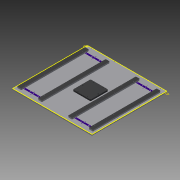
# Autodesk Inventor part: Top_part
Saved by Autodesk Inventor 2015 SP2 (Build 190223200, 223)
## iProperties
Created: 2016-11-11
Part Number: Top_part
Material: Generic
Document SubType Name: Modeling
Designer: Yann Cesbron
Density: 1 g/cm^3
Appearance: Default
Mass: 3815.36 g
Surface Area: 8876.44 cm^2
Volume: 3815.36 cm^3
Material: Perspex Black 9961 -10 mm
Author: Yann Cesbron
Autodesk Inventor part; units mm, degrees
ref_plane "YZ Plane" through (0, 0, 0) normal (1, 0, 0) x (0, 1, 0)
ref_plane "XZ Plane" through (0, 0, 0) normal (0, 1, 0) x (-1, 0, 0)
ref_plane "XY Plane" through (0, 0, 0) normal (0, 0, 1) x (1, 0, 0)
ref_plane "Work Plane2" through (0, 0, 0) normal (0, 0, 1) x (1, 0, 0)
sketch "Sketch2" plane through (0, 0, 0) normal (0, 0, 1) x (1, 0, 0)
  line L0 (-10, 10) -> (575, 10)
  line L1 (575, 10) -> (575, -540)
  line L2 (575, -540) -> (-10, -540)
  line L3 (-10, -540) -> (-10, 10)
  point P0 (0, 0)
  dimension "d0" = 585
  dimension "d1" = 550
  dimension "d3" = 10
  dimension "d10" = 10
  constraints: 8 end point, 2 parallel, 1 horizontal, 1 perpendicular
  measures "d0" distance of L1.end L2.end
  measures "d1" distance of L0.end L1.end
  measures "d3" distance from line of point (0, 0) L0
  measures "d10" distance from line of L3 point (0, 0)
extrude "Extrusion1" add sketch "Sketch2" along normal blind 10
sketch "Cut_out_top" plane through (0, 0, 10) normal (0, 0, 1) x (1, 0, 0)
  line L0 (340, -320) -> (250, -320)
  line L1 (245, -315) -> (245, -225)
  line L2 (250, -220) -> (340, -220)
  line L3 (345, -225) -> (345, -315)
  line L4 (345, -320) -> (245, -220) construction
  line L5 (245, -320) -> (345, -220) construction
  line L6 (575, 10) -> (-10, 10) projected
  line L7 (575, -540) -> (575, 10) projected
  line L8 (548, -510) -> (545, -510)
  line L9 (545, -510) -> (545, -30)
  line L10 (545, -30) -> (548, -30)
  line L11 (548, -30) -> (548, -510)
  line L12 (-10, -540) -> (575, -540) projected
  line L13 (173, -510) -> (170, -510)
  line L14 (170, -510) -> (170, -30)
  line L15 (170, -30) -> (173, -30)
  line L16 (173, -30) -> (173, -510)
  line L17 (17, -30) -> (20, -30)
  line L18 (20, -510) -> (17, -510)
  line L19 (17, -510) -> (17, -30)
  line L20 (20, -30) -> (20, -510)
  line L21 (392, -30) -> (395, -30)
  line L22 (395, -510) -> (392, -510)
  line L23 (392, -510) -> (392, -30)
  line L24 (395, -30) -> (395, -510)
  line L25 (-10, 10) -> (-10, -540) projected
  circle A0 centre (260, -327.5) radius 1.65
  circle A1 centre (330, -327.5) radius 1.65
  circle A2 centre (330, -212.5) radius 1.65
  circle A3 centre (260, -212.5) radius 1.65
  circle A4 centre (352.5, -270) radius 2.5
  circle A5 centre (237.5, -270) radius 2.5
  circle A6 centre (520, -496) radius 2.25
  circle A7 centre (420, -496) radius 2.25
  circle A8 centre (145, -496) radius 2.25
  circle A9 centre (45, -496) radius 2.25
  circle A10 centre (45, -44) radius 2.25
  circle A11 centre (145, -44) radius 2.25
  circle A12 centre (520, -44) radius 2.25
  circle A13 centre (420, -44) radius 2.25
  circle A14 centre (538, -481) radius 1.65
  circle A15 centre (538, -59) radius 1.65
  circle A16 centre (555, -411) radius 1.65
  circle A17 centre (538, -341) radius 1.65
  circle A18 centre (538, -199) radius 1.65
  circle A19 centre (555, -270) radius 1.65
  circle A20 centre (555, -129) radius 1.65
  circle A21 centre (402, -481) radius 1.65
  circle A22 centre (385, -411) radius 1.65
  circle A23 centre (402, -341) radius 1.65
  circle A24 centre (385, -270) radius 1.65
  circle A25 centre (402, -199) radius 1.65
  circle A26 centre (385, -129) radius 1.65
  circle A27 centre (402, -59) radius 1.65
  circle A28 centre (163, -481) radius 1.65
  circle A29 centre (180, -411) radius 1.65
  circle A30 centre (163, -341) radius 1.65
  circle A31 centre (180, -270) radius 1.65
  circle A32 centre (163, -199) radius 1.65
  circle A33 centre (180, -129) radius 1.65
  circle A34 centre (163, -59) radius 1.65
  circle A35 centre (27, -481) radius 1.65
  circle A36 centre (10, -411) radius 1.65
  circle A37 centre (27, -341) radius 1.65
  circle A38 centre (10, -270) radius 1.65
  circle A39 centre (27, -199) radius 1.65
  circle A40 centre (10, -129) radius 1.65
  circle A41 centre (27, -59) radius 1.65
  arc A42 (340, -320) -> (345, -315) centre (340, -315) ccw
  arc A43 (245, -315) -> (250, -320) centre (250, -315) ccw
  arc A44 (250, -220) -> (245, -225) centre (250, -225) ccw
  arc A45 (345, -225) -> (340, -220) centre (340, -225) ccw
  circle A46 centre (535, 5) radius 2.25
  circle A47 centre (370, 5) radius 2.25
  circle A48 centre (195, 5) radius 2.25
  circle A49 centre (30, 5) radius 2.25
  circle A50 centre (-5, -25) radius 2.25
  circle A51 centre (-5, -505) radius 2.25
  circle A52 centre (-5, -185) radius 2.25
  circle A53 centre (-5, -345) radius 2.25
  circle A54 centre (570, -25) radius 2.25
  circle A55 centre (570, -505) radius 2.25
  circle A56 centre (570, -345) radius 2.25
  circle A57 centre (570, -185) radius 2.25
  point P0 (0, 0)
  point P1 (295, -270)
  dimension "d6" = 100
  dimension "d7" = 100
  dimension "d8" = 280
  dimension "d9" = 280
  dimension "d49" = 3
  dimension "d50" = 480
  dimension "d53" = 3
  dimension "d54" = 480
  dimension "d55" = 3
  dimension "d56" = 480
  dimension "d57" = 3
  dimension "d58" = 480
  dimension "d59" = 30
  dimension "d60" = 30
  dimension "d61" = 30
  dimension "d62" = 150
  dimension "d63" = 30
  dimension "d64" = 30
  dimension "d65" = 30
  dimension "d66" = 150
  dimension "d94" = 3.3
  dimension "d95" = 3.3
  dimension "d96" = 3.3
  dimension "d97" = 3.3
  dimension "d98" = 15
  dimension "d99" = 15
  dimension "d100" = 15
  dimension "d101" = 15
  dimension "d102" = 7.5
  dimension "d103" = 7.5
  dimension "d104" = 7.5
  dimension "d105" = 7.5
  dimension "d106" = 245
  dimension "d111" = 5
  dimension "d112" = 5
  dimension "d113" = 7.5
  dimension "d114" = 7.5
  dimension "d115" = 50
  dimension "d116" = 50
  dimension "d132" = 4.5
  dimension "d133" = 4.5
  dimension "d134" = 4.5
  dimension "d135" = 4.5
  dimension "d136" = 4.5
  dimension "d137" = 4.5
  dimension "d138" = 4.5
  dimension "d139" = 4.5
  dimension "d147" = 55
  dimension "d148" = 44
  dimension "d149" = 44
  dimension "d150" = 100
  dimension "d151" = 55
  dimension "d152" = 44
  dimension "d153" = 100
  dimension "d154" = 44
  dimension "d155" = 54
  dimension "d156" = 54
  dimension "d157" = 55
  dimension "d158" = 100
  dimension "d159" = 55
  dimension "d160" = 54
  dimension "d161" = 54
  dimension "d162" = 100
  dimension "d163" = 3.3
  constraints: 58 centre point, 44 end point, 10 parallel, 8 point on circle, 8 point on line, 8 tangent, 5 horizontal, 5 perpendicular, 2 equal radius, 2 midpoint
  measures "d6" distance of L4.end L5.end
  measures "d7" distance of L5.start L4.end
  measures "d8" distance from line of L6 point (295, -270)
  measures "d9" distance from line of L7 point (295, -270)
  measures "d49" distance of L9.end L10.end
  measures "d50" distance of L8.end L9.end
  measures "d53" distance of L15.start L15.end
  measures "d54" distance of L13.end L15.start
  measures "d55" distance of L17.start L17.end
  measures "d56" distance of L19.start L17.start
  measures "d57" distance of L21.start L21.end
  measures "d58" distance of L23.start L21.start
  measures "d59" distance between parallel lines of L7 L9
  measures "d60" distance between parallel lines of L12 L8
  measures "d61" distance between parallel lines of L12 L22
  measures "d62" distance between parallel lines of L24 L9
  measures "d63" distance between parallel lines of L12 L18
  measures "d64" distance between parallel lines of L25 L20
  measures "d65" distance between parallel lines of L12 L13
  measures "d66" distance between parallel lines of L14 L20
  measures "d94" diameter of A0
  measures "d95" diameter of A1
  measures "d96" diameter of A2
  measures "d97" diameter of A3
  measures "d98" distance from line of L1 A0.centre
  measures "d99" distance from line of L3 A1.centre
  measures "d100" distance from line of L1 A3.centre
  measures "d101" distance from line of L3 A2.centre
  measures "d102" distance from line of L0 A1.centre
  measures "d103" distance from line of L0 A0.centre
  measures "d104" distance from line of L2 A3.centre
  measures "d105" distance from line of L2 A2.centre
  measures "d106" distance from line of L7 A1.centre
  measures "d111" diameter of A4
  measures "d112" diameter of A5
  measures "d113" distance from line of L3 A4.centre
  measures "d114" distance from line of L1 A5.centre
  measures "d115" distance from line of L0 A4.centre
  measures "d116" distance from line of L0 A5.centre
  measures "d132" diameter of A6
  measures "d133" diameter of A7
  measures "d134" diameter of A8
  measures "d135" diameter of A9
  measures "d136" diameter of A10
  measures "d137" diameter of A11
  measures "d138" diameter of A12
  measures "d139" diameter of A13
  measures "d147" distance from line of L7 A6.centre
  measures "d148" distance from line of L12 A6.centre
  measures "d149" distance from line of L12 A7.centre
  measures "d150" distance of A6.centre A7.centre
  measures "d151" distance from line of L25 A9.centre
  measures "d152" distance from line of L12 A9.centre
  measures "d153" distance of A8.centre A9.centre
  measures "d154" distance from line of L12 A8.centre
  measures "d155" distance from line of L6 A10.centre
  measures "d156" distance from line of L6 A11.centre
  measures "d157" distance from line of L25 A10.centre
  measures "d158" distance of A11.centre A10.centre
  measures "d159" distance from line of L7 A12.centre
  measures "d160" distance from line of L6 A13.centre
  measures "d161" distance from line of L6 A12.centre
  measures "d162" distance of A13.centre A12.centre
  measures "d163" diameter of A14
sketch "Air_duct_attachment_top" plane through (0, 0, 10) normal (0, 0, 1) x (1, 0, 0)
  line L0 (545, -500) -> (395, -500)
  line L1 (395, -500) -> (395, -492)
  line L2 (395, -492) -> (545, -492)
  line L3 (545, -492) -> (545, -500)
  line L4 (420, -496) -> (520, -496)
  circle A0 centre (520, -496) radius 1.65
  circle A1 centre (420, -496) radius 1.65
  line L5 (575, -540) -> (575, 10) projected
  line L6 (170, -500) -> (20, -500)
  line L7 (20, -500) -> (20, -492)
  line L8 (20, -492) -> (170, -492)
  line L9 (170, -492) -> (170, -500)
  line L10 (45, -496) -> (145, -496)
  circle A2 centre (145, -496) radius 1.65
  circle A3 centre (45, -496) radius 1.65
  line L11 (-10, -540) -> (575, -540) projected
  line L12 (545, -48) -> (395, -48)
  line L13 (395, -48) -> (395, -40)
  line L14 (395, -40) -> (545, -40)
  line L15 (545, -40) -> (545, -48)
  line L16 (420, -44) -> (520, -44)
  circle A4 centre (520, -44) radius 1.65
  circle A5 centre (420, -44) radius 1.65
  line L17 (170, -40) -> (170, -48)
  circle A6 centre (145, -44) radius 1.65
  line L18 (45, -44) -> (145, -44)
  line L19 (170, -48) -> (20, -48)
  line L20 (20, -40) -> (170, -40)
  circle A7 centre (45, -44) radius 1.65
  line L21 (20, -48) -> (20, -40)
  line L22 (-10, -540) -> (-10, 10) projected
  line L23 (575, 10) -> (-10, 10) projected
  point P0 (0, 0)
  point P1 (470, -496)
  point P2 (470, -496)
  point P3 (95, -496)
  point P4 (95, -496)
  point P5 (470, -44)
  point P6 (470, -44)
  point P7 (95, -44)
  point P8 (95, -44)
  dimension "d11" = 150
  dimension "d12" = 8
  dimension "d15" = 100
  dimension "d20" = 3.3
  dimension "d21" = 25
  dimension "d23" = 3.3
  dimension "d24" = 105
  dimension "d25" = 150
  dimension "d26" = 8
  dimension "d27" = 100
  dimension "d28" = 3.3
  dimension "d29" = 25
  dimension "d30" = 3.3
  dimension "d32" = 40
  dimension "d33" = 150
  dimension "d34" = 8
  dimension "d35" = 100
  dimension "d36" = 3.3
  dimension "d37" = 25
  dimension "d38" = 3.3
  dimension "d39" = 150
  dimension "d40" = 8
  dimension "d41" = 100
  dimension "d42" = 3.3
  dimension "d43" = 25
  dimension "d44" = 3.3
  dimension "d45" = 40
  dimension "d46" = 105
  dimension "d47" = 105
  dimension "d48" = 105
  dimension "d68" = 50
  dimension "d69" = 50
  constraints: 40 end point, 12 coincident, 12 parallel, 8 centre point, 4 horizontal, 4 midpoint, 4 perpendicular, 4 other
  measures "d11" distance of L1.end L2.end
  measures "d12" distance of L0.end L1.end
  measures "d15" distance of L4.end L4.start
  measures "d20" diameter of A1
  measures "d21" distance from line of L3 L4.end
  measures "d23" diameter of A0
  measures "d24" distance from line of L5 point (470, -496)
  measures "d25" distance of L7.end L8.end
  measures "d26" distance of L6.end L7.end
  measures "d27" distance of L10.end L10.start
  measures "d28" diameter of A3
  measures "d29" distance from line of L9 L10.end
  measures "d30" diameter of A2
  measures "d32" distance between parallel lines of L11 L0
  measures "d33" distance of L14.start L15.start
  measures "d34" distance of L12.end L14.start
  measures "d35" distance of L16.end L16.start
  measures "d36" diameter of A5
  measures "d37" distance from line of L15 L16.end
  measures "d38" diameter of A4
  measures "d39" distance of L20.start L20.end
  measures "d40" distance of L19.end L20.start
  measures "d41" distance of L18.end L18.start
  measures "d42" diameter of A7
  measures "d43" distance from line of L17 L18.end
  measures "d44" diameter of A6
  measures "d45" distance between parallel lines of L11 L6
  measures "d46" distance from line of L22 point (95, -496)
  measures "d47" distance from line of L22 point (95, -44)
  measures "d48" distance from line of L5 point (470, -44)
  measures "d68" distance between parallel lines of L23 L14
  measures "d69" distance between parallel lines of L23 L20
sketch "Flanges_top" plane through (0, 0, 10) normal (0, 0, 1) x (1, 0, 0)
  line L0 (235, -335) -> (355, -335)
  line L1 (360, -330) -> (360, -210)
  line L2 (355, -205) -> (235, -205)
  line L3 (230, -210) -> (230, -330)
  line L4 (230, -335) -> (360, -205) construction
  line L5 (360, -335) -> (230, -205) construction
  line L6 (575, -540) -> (575, 10) projected
  line L7 (575, 10) -> (-10, 10) projected
  line L8 (181.5, -520) -> (161.5, -520)
  line L9 (156.5, -515) -> (156.5, -25)
  line L10 (161.5, -20) -> (181.5, -20)
  line L11 (186.5, -25) -> (186.5, -515)
  line L12 (-10, -540) -> (575, -540) projected
  line L13 (556.5, -520) -> (536.5, -520)
  line L14 (531.5, -515) -> (531.5, -25)
  line L15 (536.5, -20) -> (556.5, -20)
  line L16 (561.5, -25) -> (561.5, -515)
  line L17 (403.5, -520) -> (383.5, -520)
  line L18 (378.5, -515) -> (378.5, -25)
  line L19 (383.5, -20) -> (403.5, -20)
  line L20 (408.5, -25) -> (408.5, -515)
  line L21 (28.5, -520) -> (8.5, -520)
  line L22 (3.5, -515) -> (3.5, -25)
  line L23 (8.5, -20) -> (28.5, -20)
  line L24 (33.5, -25) -> (33.5, -515)
  line L25 (-10, 10) -> (-10, -540) projected
  circle A0 centre (330, -327.5) radius 2.25
  circle A1 centre (260, -327.5) radius 2.25
  circle A2 centre (260, -212.5) radius 2.25
  circle A3 centre (330, -212.5) radius 2.25
  circle A4 centre (352.5, -270) radius 3.5
  circle A5 centre (237.5, -270) radius 3.5
  circle A6 centre (538, -481) radius 2.25
  circle A7 centre (538, -341) radius 2.25
  circle A8 centre (555, -411) radius 2.25
  circle A9 centre (555, -270) radius 2.25
  circle A10 centre (538, -199) radius 2.25
  circle A11 centre (555, -129) radius 2.25
  circle A12 centre (538, -59) radius 2.25
  circle A13 centre (402, -59) radius 2.25
  circle A14 centre (385, -129) radius 2.25
  circle A15 centre (402, -199) radius 2.25
  circle A16 centre (385, -270) radius 2.25
  circle A17 centre (402, -341) radius 2.25
  circle A18 centre (385, -411) radius 2.25
  circle A19 centre (402, -481) radius 2.25
  circle A20 centre (163, -481) radius 2.25
  circle A21 centre (27, -481) radius 2.25
  circle A22 centre (10, -411) radius 2.25
  circle A23 centre (180, -411) radius 2.25
  circle A24 centre (163, -341) radius 2.25
  circle A25 centre (27, -341) radius 2.25
  circle A26 centre (180, -270) radius 2.25
  circle A27 centre (10, -270) radius 2.25
  circle A28 centre (27, -199) radius 2.25
  circle A29 centre (163, -199) radius 2.25
  circle A30 centre (180, -129) radius 2.25
  circle A31 centre (163, -59) radius 2.25
  circle A32 centre (10, -129) radius 2.25
  circle A33 centre (27, -59) radius 2.25
  arc A34 (355, -335) -> (360, -330) centre (355, -330) ccw
  arc A35 (230, -330) -> (235, -335) centre (235, -330) ccw
  arc A36 (235, -205) -> (230, -210) centre (235, -210) ccw
  arc A37 (360, -210) -> (355, -205) centre (355, -210) ccw
  arc A38 (403.5, -520) -> (408.5, -515) centre (403.5, -515) ccw
  arc A39 (378.5, -515) -> (383.5, -520) centre (383.5, -515) ccw
  arc A40 (531.5, -515) -> (536.5, -520) centre (536.5, -515) ccw
  arc A41 (556.5, -520) -> (561.5, -515) centre (556.5, -515) ccw
  arc A42 (181.5, -520) -> (186.5, -515) centre (181.5, -515) ccw
  arc A43 (156.5, -515) -> (161.5, -520) centre (161.5, -515) ccw
  arc A44 (28.5, -520) -> (33.5, -515) centre (28.5, -515) ccw
  arc A45 (3.5, -515) -> (8.5, -520) centre (8.5, -515) ccw
  arc A46 (8.5, -20) -> (3.5, -25) centre (8.5, -25) ccw
  arc A47 (33.5, -25) -> (28.5, -20) centre (28.5, -25) ccw
  arc A48 (161.5, -20) -> (156.5, -25) centre (161.5, -25) ccw
  arc A49 (186.5, -25) -> (181.5, -20) centre (181.5, -25) ccw
  arc A50 (561.5, -25) -> (556.5, -20) centre (556.5, -25) ccw
  arc A51 (536.5, -20) -> (531.5, -25) centre (536.5, -25) ccw
  arc A52 (408.5, -25) -> (403.5, -20) centre (403.5, -25) ccw
  arc A53 (383.5, -20) -> (378.5, -25) centre (383.5, -25) ccw
  point P0 (0, 0)
  point P1 (295, -270)
  point P2 (156.5, -20)
  point P3 (156.5, -520)
  point P4 (186.5, -20)
  point P5 (531.5, -20)
  point P6 (531.5, -520)
  point P7 (561.5, -20)
  point P8 (378.5, -20)
  point P9 (378.5, -520)
  point P10 (408.5, -20)
  point P11 (3.5, -20)
  point P12 (3.5, -520)
  point P13 (33.5, -20)
  dimension "d70" = 130
  dimension "d72" = 280
  dimension "d73" = 280
  dimension "d74" = 130
  dimension "d75" = 30
  dimension "d76" = 500
  dimension "d78" = 30
  dimension "d79" = 500
  dimension "d82" = 30
  dimension "d83" = 500
  dimension "d84" = 30
  dimension "d85" = 500
  dimension "d86" = 20
  dimension "d87" = 20
  dimension "d88" = 20
  dimension "d89" = 20
  dimension "d90" = 13.5
  dimension "d91" = 123
  dimension "d92" = 13.5
  dimension "d93" = 123
  dimension "d107" = 4.5
  dimension "d108" = 4.5
  dimension "d109" = 4.5
  dimension "d110" = 4.5
  dimension "d117" = 7.5
  dimension "d118" = 30
  dimension "d119" = 7.5
  dimension "d120" = 30
  dimension "d121" = 7.5
  dimension "d122" = 7.5
  dimension "d123" = 30
  dimension "d124" = 30
  dimension "d126" = 7
  dimension "d127" = 7
  dimension "d128" = 65
  dimension "d129" = 65
  dimension "d130" = 7.5
  dimension "d131" = 7.5
  dimension "d257" = 4.5
  dimension "d258" = 4.5
  dimension "d259" = 4.5
  dimension "d260" = 4.5
  dimension "d261" = 4.5
  dimension "d262" = 4.5
  dimension "d263" = 4.5
  dimension "d264" = 4.5
  dimension "d265" = 4.5
  dimension "d266" = 4.5
  dimension "d267" = 4.5
  dimension "d268" = 4.5
  dimension "d269" = 4.5
  dimension "d270" = 4.5
  dimension "d271" = 4.5
  dimension "d272" = 4.5
  dimension "d273" = 4.5
  dimension "d274" = 4.5
  dimension "d275" = 4.5
  dimension "d276" = 4.5
  dimension "d277" = 4.5
  dimension "d278" = 4.5
  dimension "d279" = 4.5
  dimension "d280" = 4.5
  dimension "d281" = 4.5
  dimension "d282" = 4.5
  constraints: 54 centre point, 44 end point, 40 point on circle, 40 tangent, 32 point on line, 19 equal radius, 10 parallel, 5 horizontal, 5 perpendicular, 2 midpoint
  measures "d70" distance of L5.end L4.end
  measures "d72" distance from line of L6 point (295, -270)
  measures "d73" distance from line of L7 point (295, -270)
  measures "d74" distance between parallel lines of L0 L2
  measures "d75" distance of point (156.5, -20) point (186.5, -20)
  measures "d76" distance of point (156.5, -520) point (156.5, -20)
  measures "d78" distance of point (531.5, -20) point (561.5, -20)
  measures "d79" distance of point (531.5, -520) point (531.5, -20)
  measures "d82" distance of point (378.5, -20) point (408.5, -20)
  measures "d83" distance of point (378.5, -520) point (378.5, -20)
  measures "d84" distance of point (3.5, -20) point (33.5, -20)
  measures "d85" distance of point (3.5, -520) point (3.5, -20)
  measures "d86" distance between parallel lines of L12 L13
  measures "d87" distance between parallel lines of L12 L17
  measures "d88" distance between parallel lines of L12 L8
  measures "d89" distance between parallel lines of L12 L21
  measures "d90" distance between parallel lines of L6 L16
  measures "d91" distance between parallel lines of L14 L20
  measures "d92" distance between parallel lines of L25 L22
  measures "d93" distance between parallel lines of L9 L24
  measures "d107" diameter of A0
  measures "d108" diameter of A1
  measures "d109" diameter of A2
  measures "d110" diameter of A3
  measures "d117" distance from line of L2 A3.centre
  measures "d118" distance from line of L1 A3.centre
  measures "d119" distance from line of L2 A2.centre
  measures "d120" distance from line of L3 A2.centre
  measures "d121" distance from line of L0 A1.centre
  measures "d122" distance from line of L0 A0.centre
  measures "d123" distance from line of L1 A0.centre
  measures "d124" distance from line of L3 A1.centre
  measures "d126" diameter of A4
  measures "d127" diameter of A5
  measures "d128" distance from line of L2 A5.centre
  measures "d129" distance from line of L2 A4.centre
  measures "d130" distance from line of L1 A4.centre
  measures "d131" distance from line of L3 A5.centre
  measures "d257" diameter of A6
  measures "d258" diameter of A7
  measures "d259" diameter of A8
  measures "d260" diameter of A9
  measures "d261" diameter of A10
  measures "d262" diameter of A11
  measures "d263" diameter of A12
  measures "d264" diameter of A13
  measures "d265" diameter of A14
  measures "d266" diameter of A15
  measures "d267" diameter of A16
  measures "d268" diameter of A17
  measures "d269" diameter of A18
  measures "d270" diameter of A19
  measures "d271" diameter of A20
  measures "d272" diameter of A21
  measures "d273" diameter of A22
  measures "d274" diameter of A23
  measures "d275" diameter of A24
  measures "d276" diameter of A25
  measures "d277" diameter of A26
  measures "d278" diameter of A27
  measures "d279" diameter of A28
  measures "d280" diameter of A29
  measures "d281" diameter of A30
  measures "d282" diameter of A31
sketch "Panel_back_holes_top" plane through (-10, -540, 0) normal (0, -1, 0) x (1, 0, 0)
  circle A0 centre (40, 5) radius 1.65
  circle A1 centre (205, 5) radius 1.65
  circle A2 centre (380, 5) radius 1.65
  circle A3 centre (545, 5) radius 1.65
  line L0 (0, 10) -> (585, 10) projected
  line L1 (585, 0) -> (585, 10) projected
  line L2 (0, 0) -> (0, 10) projected
  point P0 (10, 0)
  dimension "d356" = 3.3
  dimension "d357" = 3.3
  dimension "d358" = 3.3
  dimension "d359" = 3.3
  dimension "d360" = 5
  dimension "d361" = 40
  dimension "d362" = 5
  dimension "d363" = 5
  dimension "d364" = 40
  dimension "d365" = 5
  dimension "d366" = 165
  dimension "d367" = 165
  constraints: 4 centre point
  measures "d356" diameter of A0
  measures "d357" diameter of A1
  measures "d358" diameter of A2
  measures "d359" diameter of A3
  measures "d360" distance from line of L0 A3.centre
  measures "d361" distance from line of L1 A3.centre
  measures "d362" distance from line of L0 A2.centre
  measures "d363" distance from line of L0 A0.centre
  measures "d364" distance from line of L2 A0.centre
  measures "d365" distance from line of L0 A1.centre
  measures "d366" distance of A1.centre A0.centre
  measures "d367" distance of A2.centre A3.centre
extrude "Extrusion2" cut sketch "Cut_out_top" against normal blind 10 keep common part
extrude "Extrusion3" add sketch "Flanges_top" along normal blind 10 separate body contours A35 L3 A36 L2 A37 L1 A34 L0
extrude "Extrusion4" cut sketch "Panel_back_holes_top" against normal blind 15 bodies 1
extrude "Extrusion5" add sketch "Flanges_top" along normal blind 10 separate body contours L13 A40 L14 A51 L15 A50 L16 A41
extrude "Extrusion6" add sketch "Flanges_top" along normal blind 10 separate body contours L17 A39 L18 A53 L19 A52 L20 A38
extrude "Extrusion7" add sketch "Flanges_top" along normal blind 10 separate body contours L8 A43 L9 A48 L10 A49 L11 A42
extrude "Extrusion8" add sketch "Flanges_top" along normal blind 10 separate body contours L21 A45 L22 A46 L23 A47 L24 A44
